Autodesk Inventor part; units mm, degrees
(part 2 of 2)
  line L96 (-51.9611, 31.9) -> (-49.3079, 31.9)
  line L97 (-49.3079, 31.9) -> (-49.3079, 31.5789)
  line L98 (-49.3079, 31.5789) -> (-51.9611, 31.5789)
  spline S110 degree 2 poles (-51.7594, 30.0454) (-51.7882, 30.0846) (-51.8911, 30.2163) (-51.922, 30.278) knots 0 0 0 1 2 2 2
  spline S111 degree 2 poles (-51.922, 30.278) (-51.9673, 30.3624) (-52.0146, 30.5209) (-52.0146, 30.665) knots 0 0 0 1 2 2 2
  spline S112 degree 2 poles (-52.0146, 30.665) (-52.0146, 30.7823) (-51.9261, 30.9943) (-51.8459, 31.0746) knots 0 0 0 1 2 2 2
  spline S113 degree 2 poles (-51.8459, 31.0746) (-51.7676, 31.1508) (-51.5371, 31.2434) (-51.4095, 31.2434) knots 0 0 0 1 2 2 2
  spline S114 degree 2 poles (-51.4095, 31.2434) (-51.2119, 31.2434) (-50.932, 31.0767) (-50.8517, 30.8955) knots 0 0 0 1 2 2 2
  spline S115 degree 2 poles (-50.8517, 30.8955) (-50.7776, 30.735) (-50.722, 30.2986) (-50.7076, 30.0454) knots 0 0 0 1 2 2 2
  line L99 (-50.7076, 30.0454) -> (-50.6458, 30.0454)
  spline S116 degree 2 poles (-50.6458, 30.0454) (-50.5347, 30.0454) (-50.3968, 30.1134) (-50.3577, 30.1751) knots 0 0 0 1 2 2 2
  spline S117 degree 2 poles (-50.3577, 30.1751) (-50.3186, 30.2369) (-50.2939, 30.4139) (-50.2939, 30.5086) knots 0 0 0 1 2 2 2
  spline S118 degree 2 poles (-50.2939, 30.5086) (-50.2939, 30.6197) (-50.3597, 30.9202) (-50.4235, 31.0705) knots 0 0 0 1 2 2 2
  line L100 (-50.4235, 31.0705) -> (-50.4235, 31.089)
  line L101 (-50.4235, 31.089) -> (-50.0963, 31.089)
  spline S119 degree 2 poles (-50.0963, 31.089) (-50.0716, 31.0005) (-50.0098, 30.6691) (-50.0098, 30.5065) knots 0 0 0 1 2 2 2
  spline S120 degree 2 poles (-50.0098, 30.5065) (-50.0098, 30.3089) (-50.0716, 30.0393) (-50.1518, 29.9322) knots 0 0 0 1 2 2 2
  spline S121 degree 2 poles (-50.1518, 29.9322) (-50.2301, 29.8273) (-50.4791, 29.7243) (-50.6582, 29.7243) knots 0 0 0 1 2 2 2
  line L102 (-50.6582, 29.7243) -> (-51.9611, 29.7243)
  line L103 (-51.9611, 29.7243) -> (-51.9611, 30.0454)
  line L104 (-51.9611, 30.0454) -> (-51.7594, 30.0454)
  line L105 (-51.4918, 30.0454) -> (-50.9628, 30.0454)
  spline S122 degree 2 poles (-50.9628, 30.0454) (-50.9731, 30.1607) (-51.0081, 30.5086) (-51.041, 30.6177) knots 0 0 0 1 2 2 2
  spline S123 degree 2 poles (-51.041, 30.6177) (-51.0802, 30.7453) (-51.2428, 30.912) (-51.3868, 30.912) knots 0 0 0 1 2 2 2
  spline S124 degree 2 poles (-51.3868, 30.912) (-51.5515, 30.912) (-51.7182, 30.7268) (-51.7182, 30.5497) knots 0 0 0 1 2 2 2
  spline S125 degree 2 poles (-51.7182, 30.5497) (-51.7182, 30.3995) (-51.5886, 30.1525) (-51.4918, 30.0454) knots 0 0 0 1 2 2 2
  line L106 (-51.9611, 27.7771) -> (-51.9611, 28.0982)
  line L107 (-51.9611, 28.0982) -> (-50.8743, 28.0982)
  spline S126 degree 2 poles (-50.8743, 28.0982) (-50.7426, 28.0982) (-50.5162, 28.123) (-50.4482, 28.16) knots 0 0 0 1 2 2 2
  spline S127 degree 2 poles (-50.4482, 28.16) (-50.3762, 28.1991) (-50.3062, 28.3391) (-50.3062, 28.4585) knots 0 0 0 1 2 2 2
  spline S128 degree 2 poles (-50.3062, 28.4585) (-50.3062, 28.5778) (-50.4338, 28.831) (-50.5367, 28.9525) knots 0 0 0 1 2 2 2
  line L108 (-50.5367, 28.9525) -> (-51.9611, 28.9525)
  line L109 (-51.9611, 28.9525) -> (-51.9611, 29.2736)
  line L110 (-51.9611, 29.2736) -> (-50.0551, 29.2736)
  line L111 (-50.0551, 29.2736) -> (-50.0551, 28.9525)
  line L112 (-50.0551, 28.9525) -> (-50.2671, 28.9525)
  spline S129 degree 2 poles (-50.2671, 28.9525) (-50.1374, 28.8084) (-50.0016, 28.5305) (-50.0016, 28.3741) knots 0 0 0 1 2 2 2
  spline S130 degree 2 poles (-50.0016, 28.3741) (-50.0016, 28.0941) (-50.3721, 27.7771) (-50.7241, 27.7771) knots 0 0 0 1 2 2 2
  line L113 (-50.7241, 27.7771) -> (-51.9611, 27.7771)
  line L114 (-51.9611, 25.7476) -> (-51.9611, 26.1696)
  line L115 (-51.9611, 26.1696) -> (-51.041, 26.8777)
  line L116 (-51.041, 26.8777) -> (-51.1645, 27.0053)
  line L117 (-51.1645, 27.0053) -> (-51.9611, 27.0053)
  line L118 (-51.9611, 27.0053) -> (-51.9611, 27.3264)
  line L119 (-51.9611, 27.3264) -> (-49.3079, 27.3264)
  line L120 (-49.3079, 27.3264) -> (-49.3079, 27.0053)
  line L121 (-49.3079, 27.0053) -> (-50.8599, 27.0053)
  line L122 (-50.8599, 27.0053) -> (-50.0551, 26.2519)
  line L123 (-50.0551, 26.2519) -> (-50.0551, 25.8526)
  line L124 (-50.0551, 25.8526) -> (-50.8517, 26.6348)
  line L125 (-50.8517, 26.6348) -> (-51.9611, 25.7476)
  point P0 (0, 0)
  dimension "d79" = 17
  dimension "d80" = 17
  dimension "d81" = 8
  dimension "d82" = 12
  dimension "d83" = 16
  dimension "d86" = 9
  constraints: 12 centre point, 10 equal radius, 6 coincident, 4 vertical alignment, 3 point on line, 2 end point, 2 horizontal alignment, 1 horizontal, 10 other
  measures "d79" distance of A3.centre A4.centre
  measures "d80" distance of A5.centre A4.centre
  measures "d81" diameter of A3
  measures "d82" distance of A0.centre A3.centre
  measures "d83" distance from line of L3 A3.centre
  measures "d86" diameter of A6
emboss "Emboss1" sketch "Sketch2" operation cut depth 0.01 direction (0, 1, 0)
body "Solid1"
